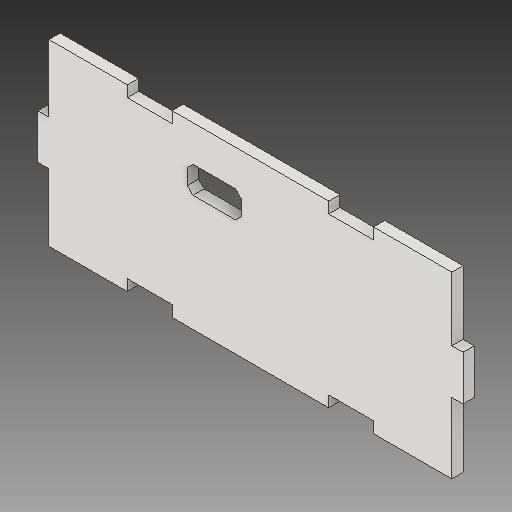
# Autodesk Inventor part: side
Saved by Autodesk Inventor 2018.2 (Build 222227000, 227)
## iProperties
Created: 2018-04-16
Part Number: side
Material: ABS Plastic
Document SubType Name: Modeling
Designer: Derek Fronek
Density: 1.06 g/cm^3
Appearance: Smooth - White
Author: Derek Fronek
Autodesk Inventor part; units mm, degrees
ref_plane "YZ Plane" through (0, 0, 0) normal (1, 0, 0) x (0, 1, 0)
ref_plane "XZ Plane" through (0, 0, 0) normal (0, 1, 0) x (-1, 0, 0)
ref_plane "XY Plane" through (0, 0, 0) normal (0, 0, 1) x (1, 0, 0)
sketch "Sketch1" plane through (0, 0, 0) normal (0, 0, 1) x (1, 0, 0)
  line L0 (22.225, 3.175) -> (25.4, 3.175) projected
  line L1 (-37.5498, -13.069) -> (-39.1373, -14.6565) projected
  line L2 (-39.1373, -14.6565) -> (-51.2023, -14.6565) projected
  line L3 (-51.2023, -14.6565) -> (-52.7898, -13.069) projected
  line L4 (-52.7898, -13.069) -> (-52.7898, -8.624) projected
  line L5 (-52.7898, -8.624) -> (-51.2023, -7.0365) projected
  line L6 (-51.2023, -7.0365) -> (-39.1373, -7.0365) projected
  line L7 (-39.1373, -7.0365) -> (-37.5498, -8.624) projected
  line L8 (-37.5498, -8.624) -> (-37.5498, -13.069) projected
  line L9 (-95.25, 3.175) -> (-95.25, -15.875) projected
  line L10 (-95.25, -28.575) -> (-95.25, -47.625) projected
  line L11 (-95.25, -47.625) -> (-69.85, -47.625) projected
  line L12 (-69.85, -47.625) -> (-69.85, -44.45) projected
  line L13 (-69.85, -44.45) -> (-57.15, -44.45) projected
  line L14 (-57.15, -44.45) -> (-57.15, -47.625) projected
  line L15 (-57.15, -47.625) -> (-12.7, -47.625) projected
  line L16 (-12.7, -47.625) -> (-12.7, -44.45) projected
  line L17 (-12.7, -44.45) -> (0, -44.45) projected
  line L18 (0, -44.45) -> (0, -47.625) projected
  line L19 (22.225, 3.175) -> (0, 3.175)
  line L20 (0, 3.175) -> (0, 0)
  line L21 (0, 0) -> (-12.7, 0)
  line L22 (-12.7, 0) -> (-12.7, 3.175)
  line L23 (-12.7, 3.175) -> (-57.15, 3.175)
  line L24 (-57.15, 3.175) -> (-57.15, 0)
  line L25 (-57.15, 0) -> (-69.85, 0)
  line L26 (-69.85, 0) -> (-69.85, 3.175)
  line L27 (-69.85, 3.175) -> (-95.25, 3.175)
  line L28 (-48.8955, -19.685) -> (-50.483, -21.2725) projected
  line L29 (-50.483, -21.2725) -> (-63.3813, -21.2725) projected
  line L30 (-63.3813, -21.2725) -> (-64.9688, -19.685) projected
  line L31 (-64.9688, -19.685) -> (-64.9688, -10.4775) projected
  line L32 (-64.9688, -10.4775) -> (-63.3813, -8.89) projected
  line L33 (-63.3813, -8.89) -> (-50.483, -8.89) projected
  line L34 (-50.483, -8.89) -> (-48.8955, -10.4775) projected
  line L35 (-48.8955, -10.4775) -> (-48.8955, -19.685) projected
  line L36 (0, 0) -> (0, 3.175) projected
  line L37 (-12.7, 0) -> (0, 0) projected
  line L38 (-12.7, 3.175) -> (-12.7, 0) projected
  line L39 (-57.15, 3.175) -> (-12.7, 3.175) projected
  line L40 (-57.15, 0) -> (-57.15, 3.175) projected
  line L41 (-69.85, 0) -> (-57.15, 0) projected
  line L42 (-69.85, 3.175) -> (-69.85, 0) projected
  line L43 (-92.075, 3.175) -> (-69.85, 3.175) projected
  line L44 (-92.075, -15.875) -> (-92.075, 3.175) projected
  line L45 (-95.25, -15.875) -> (-92.075, -15.875) projected
  line L46 (-95.25, -28.575) -> (-95.25, -15.875) projected
  line L47 (-92.075, -28.575) -> (-95.25, -28.575) projected
  line L48 (-92.075, -47.625) -> (-92.075, -28.575) projected
  line L49 (-69.85, -47.625) -> (-92.075, -47.625) projected
  line L50 (-69.85, -44.45) -> (-69.85, -47.625) projected
  line L51 (-57.15, -44.45) -> (-69.85, -44.45) projected
  line L52 (-57.15, -47.625) -> (-57.15, -44.45) projected
  line L53 (-12.7, -47.625) -> (-57.15, -47.625) projected
  line L54 (-12.7, -44.45) -> (-12.7, -47.625) projected
  line L55 (0, -44.45) -> (-12.7, -44.45) projected
  line L56 (0, -47.625) -> (0, -44.45) projected
  line L57 (22.225, -47.625) -> (0, -47.625) projected
  line L58 (22.225, -27.6225) -> (22.225, -47.625) projected
  line L59 (25.4, -27.6225) -> (22.225, -27.6225) projected
  line L60 (25.4, -14.9225) -> (25.4, -27.6225) projected
  line L61 (22.225, -14.9225) -> (25.4, -14.9225) projected
  line L62 (22.225, 3.175) -> (22.225, -14.9225) projected
  line L63 (0, 3.175) -> (22.225, 3.175) projected
  point P0 (25.4, -15.875)
  constraints: 18 end point, 6 perpendicular, 5 point on line, 1 horizontal
extrude "Extrusion1" add sketch "Sketch1" along normal blind 3.175 contours L35 L28 L29 L30 L31 L32 L33 L4 L3 L2 | L45 L44 L27 L26 L25 L24 L23 L22 L21 L20 L19 L62 L61 L60 L59 L58 L57 L18 L17 L16 L15 L14 L13 L12 L11 L48 L47 L46
body "Solid1"
